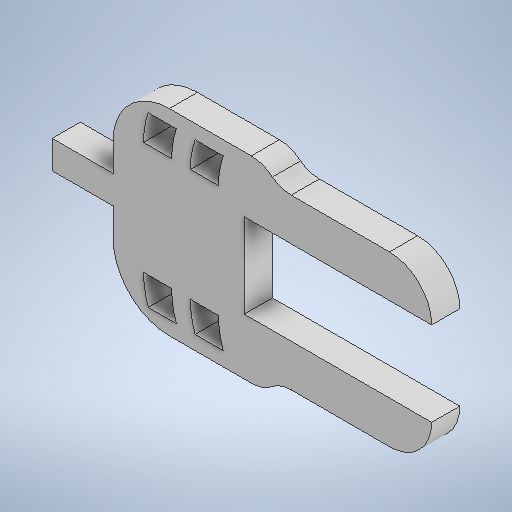
# Autodesk Inventor part: MOTOR
Saved by Autodesk Inventor 2025.1 (Build 291241000, 241)
## iProperties
Created: 2024-10-25
Part Number: MOTOR
Material: Genérico
Document SubType Name: Modeling
Designer: Aluno
Density: 1 g/cm^3
Appearance: Padrão
Author: Aluno
Autodesk Inventor part; units mm, degrees
ref_plane "YZ Plane" through (0, 0, 0) normal (1, 0, 0) x (0, 1, 0)
ref_plane "XZ Plane" through (0, 0, 0) normal (0, 1, 0) x (-1, 0, 0)
ref_plane "XY Plane" through (0, 0, 0) normal (0, 0, 1) x (1, 0, 0)
sketch "Esboço1" plane through (0, 0, 0) normal (0, 0, 1) x (1, 0, 0)
  line L0 (-6.5, 1.5) -> (-6.5, 0)
  line L1 (-6.5, 1.5) -> (0, 1.5)
  line L2 (0, 4.5) -> (0, 1.5)
  line L3 (6, 10.5) -> (14.75, 10.5)
  line L4 (14, 4.5) -> (14, 0)
  line L5 (14, 4.5) -> (34, 4.5)
  arc A0 (6, 10.5) -> (0, 4.5) centre (6, 4.5) ccw
  line L6 (14, 10.5) -> (14.75, 10.5)
  arc A1 (17, 9.6677) -> (14.75, 10.5) centre (14.75, 7.0427) ccw
  arc A2 (17, 9.6677) -> (19.0095, 9) centre (19.0095, 12.3577) ccw
  line L7 (20, 9) -> (19.0095, 9)
  line L8 (20, 9) -> (29.5, 9)
  arc A3 (34, 4.5) -> (29.5, 9) centre (29.5, 4.5) ccw
  line L9 (3.2492, 6) -> (6.2492, 6)
  arc A4 (3.7492, 9) -> (3.2492, 6) centre (12.4992, 6) ccw
  arc A5 (6.7492, 9) -> (6.2492, 6) centre (15.4992, 6) ccw
  line L10 (3.7492, 9) -> (6.7492, 9)
  line L11 (8.2492, 6) -> (11.2492, 6)
  arc A6 (8.7492, 9) -> (8.2492, 6) centre (17.4992, 6) ccw
  arc A7 (11.7492, 9) -> (11.2492, 6) centre (20.4992, 6) ccw
  line L12 (8.7492, 9) -> (11.7492, 9)
  line L13 (-6.5, -1.5) -> (-6.5, 0)
  line L14 (-6.5, -1.5) -> (0, -1.5)
  line L15 (0, -4.5) -> (0, -1.5)
  line L16 (6, -10.5) -> (14.75, -10.5)
  line L17 (14, -4.5) -> (14, 0)
  line L18 (14, -4.5) -> (34, -4.5)
  arc A8 (0, -4.5) -> (6, -10.5) centre (6, -4.5) ccw
  line L19 (14, -10.5) -> (14.75, -10.5)
  arc A9 (14.75, -10.5) -> (17, -9.6677) centre (14.75, -7.0427) ccw
  arc A10 (19.0095, -9) -> (17, -9.6677) centre (19.0095, -12.3577) ccw
  line L20 (20, -9) -> (19.0095, -9)
  line L21 (20, -9) -> (29.5, -9)
  arc A11 (29.5, -9) -> (34, -4.5) centre (29.5, -4.5) ccw
  line L22 (3.2492, -6) -> (6.2492, -6)
  arc A12 (3.2492, -6) -> (3.7492, -9) centre (12.4992, -6) ccw
  arc A13 (6.2492, -6) -> (6.7492, -9) centre (15.4992, -6) ccw
  line L23 (3.7492, -9) -> (6.7492, -9)
  arc A14 (11.2492, -6) -> (11.7492, -9) centre (20.4992, -6) ccw
  line L24 (8.7492, -9) -> (11.7492, -9)
  line L25 (8.2492, -6) -> (11.2492, -6)
  arc A15 (8.2492, -6) -> (8.7492, -9) centre (17.4992, -6) ccw
  point P0 (0, 0)
  point P1 (6.2492, -6)
  point P2 (11.2492, -6)
  point P3 (11.2492, 6)
  constraints: 52 end point, 32 point on circle, 16 centre point, 9 horizontal, 5 tangent, 2 point on line, 2 vertical
extrude "Extrusão1" add sketch "Esboço1" along normal blind 3
